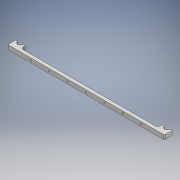
# Autodesk Inventor part: SuporteAntiEmpenamento
Saved by Autodesk Inventor 2018 (Build 220112000, 112)
## iProperties
Created: 2018-07-24
Part Number: SuporteAntiEmpenamento
Material: Genérico
Document SubType Name: Modeling
Designer: Usuario
Density: 1 g/cm^3
Appearance: Padrão
Mass: 34.9161 g
Surface Area: 151.77 cm^2
Volume: 34.9161 cm^3
Author: Usuario
Autodesk Inventor part; units mm, degrees
ref_plane "YZ Plane" through (0, 0, 0) normal (1, 0, 0) x (0, 1, 0)
ref_plane "XZ Plane" through (0, 0, 0) normal (0, 1, 0) x (-1, 0, 0)
ref_plane "XY Plane" through (0, 0, 0) normal (0, 0, 1) x (1, 0, 0)
sketch "Esboço1" plane through (0, 0, 0) normal (0, 0, 1) x (1, 0, 0)
  arc A0 (-6, 0) -> (6, 0) centre (0, 0) ccw
  arc A1 (-326, 0) -> (-314, 0) centre (-320, 0) ccw
  line L0 (10.5, 0) -> (10.5, -15)
  line L1 (-330.5, 0) -> (-330.5, -15)
  line L2 (-328.5, -17) -> (8.5, -17)
  line L3 (-10.5, 0) -> (-10.5, -4)
  line L4 (-309.5, 0) -> (-309.5, -4)
  line L5 (-303.5, -10) -> (-16.5, -10)
  line L6 (10.5, 0) -> (5.995, 0)
  line L7 (-5.995, 0) -> (-10.5, 0)
  line L8 (-309.5, 0) -> (-314.005, 0)
  line L9 (-325.995, 0) -> (-330.5, 0)
  line L10 (8.5, -17) -> (10.5, -15)
  line L11 (-328.5, -17) -> (-330.5, -15)
  arc A2 (-309.5, -4) -> (-303.5, -10) centre (-303.5, -4) ccw
  arc A3 (-16.5, -10) -> (-10.5, -4) centre (-16.5, -4) ccw
  point P0 (10.5, -17)
  point P1 (-330.5, -17)
  dimension "d1" = 12
  dimension "d2" = 12
  dimension "d5" = 2
  dimension "d6" = 2
  dimension "d7" = 2
  dimension "d8" = 2
  dimension "d9" = 6
  dimension "d29" = 7
  constraints: 24 end point, 8 point on circle, 8 point on line, 5 perpendicular, 4 centre point, 4 collinear, 4 tangent, 3 vertical, 1 equal radius
  measures "d1" diameter of A0
  measures "d2" diameter of A1
  measures "d5" distance of L2.end point (10.5, -17)
  measures "d6" distance of L0.end point (10.5, -17)
  measures "d7" distance of L2.start point (-330.5, -17)
  measures "d8" distance of L1.end point (-330.5, -17)
  measures "d9" radius of A2
  measures "d29" distance between parallel lines of L2 L5
extrude "Extrusão1" add sketch "Esboço1" against normal blind 9.52
sketch "Esboço2" plane through (-328.5, -17, 0) normal (0, -1, 0) x (1, 0, 0)
  line L0 (334.5, 0) -> (334.5, -9.52) projected
  line L1 (334.5, -4.76) -> (2.5, -4.76) construction
  line L2 (2.5, 0) -> (2.5, -9.52) projected
  circle A0 centre (168.5, -4.76) radius 2 construction
  circle A1 centre (128.5, -4.76) radius 2 construction
  circle A2 centre (88.5, -4.76) radius 2 construction
  circle A3 centre (48.5, -4.76) radius 2 construction
  circle A4 centre (208.5, -4.76) radius 2 construction
  circle A5 centre (168.5, -4.76) radius 2 construction
  circle A6 centre (128.5, -4.76) radius 2 construction
  circle A7 centre (88.5, -4.76) radius 2 construction
  circle A8 centre (248.5, -4.76) radius 2 construction
  circle A9 centre (208.5, -4.76) radius 2 construction
  circle A10 centre (168.5, -4.76) radius 2 construction
  circle A11 centre (128.5, -4.76) radius 2 construction
  circle A12 centre (288.5, -4.76) radius 2 construction
  circle A13 centre (248.5, -4.76) radius 2 construction
  circle A14 centre (208.5, -4.76) radius 2 construction
  circle A15 centre (168.5, -4.76) radius 2 construction
  point P0 (328.5, 0)
  dimension "d12" = 4
  dimension "d15" = 40
  dimension "d18" = 40
  constraints: 16 centre point, 3 midpoint, 2 end point, 2 horizontal, 30 other
  measures "d12" diameter of A0
  measures "d15" distance of A0.centre A1.centre
  measures "d18" distance of A0.centre A4.centre
hole "Furo1" at (-40, -17, -4.76) at (-80, -17, -4.76) at (-120, -17, -4.76) at (-160, -17, -4.76) at (-200, -17, -4.76) at (-240, -17, -4.76) at (-280, -17, -4.76) direction (0, 1, 0) diameter 3.242 end through all thread size "M4x0.7" class "6H" standard "ISO Metric profile"
equation "\"d6\" = d5"
equation "\"d8\" = d7"
